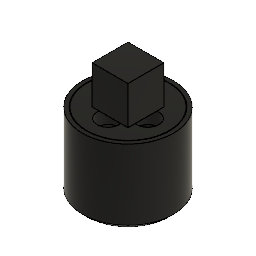
Sensor (Autodesk Fusion 360 design; units mm, degrees)
Autodesk Fusion 360 part; units mm, degrees
note: some values were not read from the file. Chosen so that the rebuilt part matches the saved one: which face or edge a step refers to; how an offset face is resized. Set by a fixed rule: which sketch regions a step uses.
sketch "Skizze1" plane through (0, 0, 0) normal (0, 0, 1) x (1, 0, 0)
  circle A0 centre (0, 0) radius 9.45
  line L0 (-4.1, 4.1) -> (4.1, 4.1)
  line L1 (4.1, 4.1) -> (4.1, -4.1)
  line L2 (4.1, -4.1) -> (-4.1, -4.1)
  line L3 (-4.1, -4.1) -> (-4.1, 4.1)
  line L4 (-4.1, 0) -> (4.1, 0) construction
  line L5 (0, 4.1) -> (0, -4.1) construction
  circle A1 centre (4.5, 0) radius 2.5
  circle A2 centre (0, 4.5) radius 2.5
  circle A3 centre (-4.5, 0) radius 2.5
  circle A4 centre (0, -4.5) radius 2.5
  circle A5 centre (0, 0) radius 7.6
  dimension "d18" = 18.9
  dimension "d19" = 8.2
  dimension "d20" = 8.2
  dimension "d21" = 5
  dimension "d22" = 4.5
  dimension "d24" = 360
  dimension "d25" = 15.2
  measures "d18" diameter of A0
  measures "d19" distance of L0.start L0.end
  measures "d20" distance of L0.start L2.end
  measures "d21" diameter of A1
  measures "d22" distance of A0.centre A1.centre
  measures "d25" diameter of A5
extrude "Extrusion1" add sketch "Skizze1" against normal blind 3 contours A0 | L0 L1 L2 L3 A1 A2 A3 A4 | A5 makes body 1
extrude "Extrusion2" add sketch "Skizze1" against normal blind 5 contours A0 bodies 1
extrude "Extrusion3" add sketch "Skizze1" along normal blind 8.7 contours L0 L1 L2 L3 A1 A2 A3 A4 | L0 A2 | L3 A3 | L1 A1 | L2 A4 picked at (-0.6822, 3.4278) picked at (-2.9892, -0.0816) picked at (3.4222, -0.6072) picked at (0.6072, -3.6626) bodies 1
sketch "Skizze2" plane through (0, 0, 0) normal (0, 0, 1) x (1, 0, 0)
  circle A0 centre (0, 0) radius 10.35
  circle A1 centre (0, 0) radius 9.35
  circle A2 centre (0, 0) radius 6.75
  circle A3 centre (0, 0) radius 1.25
  circle A4 centre (0, -4.55) radius 2.2
  line L0 (0, -4.55) -> (0, 0)
  dimension "d32" = 20.7
  dimension "d33" = 18.7
  dimension "d34" = 13.5
  dimension "d35" = 2.5
  dimension "d36" = 4.4
  measures "d32" diameter of A0
  measures "d33" diameter of A1
  measures "d34" diameter of A2
  measures "d35" diameter of A3
  measures "d36" diameter of A4
extrude "Extrusion4" add sketch "Skizze2" against normal blind 17 separate body contours A0 makes body 2
extrude "Extrusion6" add sketch "Skizze2" against normal blind 11.3 contours A1 bodies 2
extrude "Extrusion7" add sketch "Skizze2" against normal blind 3.2 contours A2 bodies 2
thread "Gewinde1" "ISO Metric profile 3.0 M3x0.5 6H" major diameter 3.086 minor diameter 2.529 pitch 0.5 angle 60 resizes the face on face at (1.2438, -0.1245, -2.1333) on bodies 2
chamfer "Fase1" distance 1 angle 45 1 edges at (-9.6496, -3.7427, 0) on bodies 2
copy_body "Körper->Berechn1" bodies 1 removing the originals makes body 3 in component "lid"
copy_body "Körper->Berechn2" bodies 2 removing the originals makes body 4 in component "body"
component "lid" placed x (1, 0, 0) y (0, 1, 0) z (0, 0, 1) at (0, 0, 0)
component "body" placed x (1, 0, 0) y (0, -1, 0) z (0, 0, -1) at (0, 0, -17)
equation "d22 = ( 14 / 2 ) * 1 mm - 2.5 mm"
equation "d41 = -17 mm + 5.7 mm"
equation "d43 = -17 mm + 13.8 mm"
